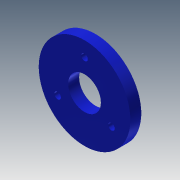
# Autodesk Inventor part: uchyt_lozisko_kruh
Saved by Autodesk Inventor 2013 (Build 170138000, 138)
## iProperties
Created: 2013-05-11
Part Number: uchyt_lozisko_kruh
Material: Generic
Document SubType Name: Modeling
Designer: idle-rug
Density: 1 g/cm^3
Author: idle-rug
Autodesk Inventor part; units mm, degrees
ref_plane "YZ Plane" through (0, 0, 0) normal (1, 0, 0) x (0, 1, 0)
ref_plane "XZ Plane" through (0, 0, 0) normal (0, 1, 0) x (-1, 0, 0)
ref_plane "XY Plane" through (0, 0, 0) normal (0, 0, 1) x (1, 0, 0)
sketch "Sketch1" plane through (0, 0, 0) normal (0, 1, 0) x (-1, 0, 0)
  circle A0 centre (0, 0) radius 21
  circle A1 centre (0, 0) radius 7.5
  line L0 (0, -7.5) -> (0, -21)
  circle A2 centre (0, 14.25) radius 1.5
  line L1 (0, 0) -> (14.25, 0) construction
  line L2 (0, 0) -> (14.25, 0) construction
  circle A3 centre (-12.3409, -7.125) radius 1.5
  line L3 (0, 0) -> (14.25, 0) construction
  circle A4 centre (12.3409, -7.125) radius 1.5
  constraints: 8 end point, 4 coincident, 3 centre point, 3 horizontal, 2 vertical alignment, 1 vertical, 4 other
extrude "Extrusion1" add sketch "Sketch1" along normal blind 5
body "Solid1"
